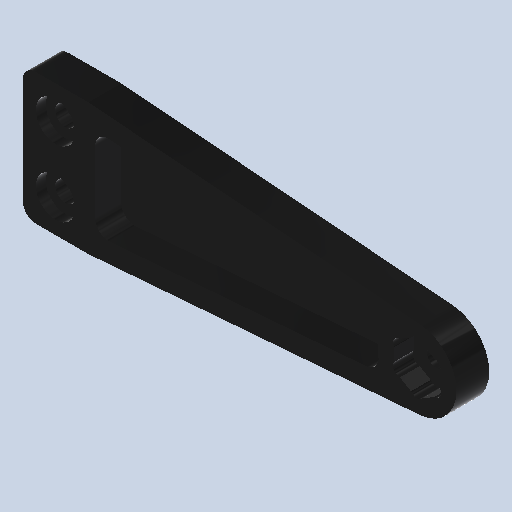
# Autodesk Inventor part: Trunk_handle_frame
Saved by Autodesk Inventor 2022.4 (Build 264492000, 492)
## iProperties
Created: 2016-05-25
Part Number: Trunk_handle_frame
Material: アセタール樹脂、黒
Document SubType Name: Modeling
Designer: hiroaki
Density: 1.425 g/cm^3
Appearance: 滑らか - 黒
Mass: 4.5833 g
Surface Area: 34.8824 cm^2
Volume: 3.21635 cm^3
Description: POM T5
Author: hiroaki
Autodesk Inventor part; units mm, degrees
ref_plane "YZ Plane" through (0, 0, 0) normal (1, 0, 0) x (0, 1, 0)
ref_plane "XZ Plane" through (0, 0, 0) normal (0, 1, 0) x (-1, 0, 0)
ref_plane "XY Plane" through (0, 0, 0) normal (0, 0, 1) x (1, 0, 0)
sketch "スケッチ1" plane through (0, 0, 0) normal (0, 0, 1) x (1, 0, 0)
  circle A0 centre (5, 5) radius 1.55
  circle A1 centre (5, -5) radius 1.55
  line L0 (0, 0) -> (60, 0) construction
  circle A2 centre (60, 0) radius 1.55
  line L1 (0, 10) -> (0, -10)
  line L2 (0, -10) -> (10, -10)
  line L3 (10, -10) -> (60.4762, -5.9811)
  line L4 (10, 10) -> (60.4762, 5.9811)
  arc A3 (60.4762, -5.9811) -> (60.4762, 5.9811) centre (60, 0) ccw
  line L5 (55.0583, -3.4029) -> (11, -6.9109)
  line L6 (55.0583, 3.4029) -> (11, 6.9109)
  arc A4 (55.0583, 3.4029) -> (55.0583, -3.4029) centre (60, 0) ccw
  line L7 (11, -6.9109) -> (11, 6.9109)
  line L8 (5, -5) -> (5, 5) construction
  line L9 (0, 10) -> (10, 10)
  line L10 (8.01, 6.7378) -> (8.01, 3.2622) construction
  line L11 (8.01, 3.2622) -> (5, 1.5244) construction
  line L12 (5, 1.5244) -> (1.99, 3.2622) construction
  line L13 (1.99, 3.2622) -> (1.99, 6.7378) construction
  line L14 (1.99, 6.7378) -> (5, 8.4756) construction
  line L15 (5, 8.4756) -> (8.01, 6.7378) construction
  arc A5 (4.0907, 2.0494) -> (5.9093, 2.0494) centre (5, 2.5744) ccw construction
  arc A6 (7.1007, 2.7372) -> (8.01, 4.3122) centre (7.1007, 3.7872) ccw construction
  arc A7 (8.01, 5.6878) -> (7.1007, 7.2628) centre (7.1007, 6.2128) ccw construction
  arc A8 (5.9093, 7.9506) -> (4.0907, 7.9506) centre (5, 7.4256) ccw construction
  arc A9 (2.8993, 7.2628) -> (1.99, 5.6878) centre (2.8993, 6.2128) ccw construction
  arc A10 (1.99, 4.3122) -> (2.8993, 2.7372) centre (2.8993, 3.7872) ccw construction
  line L16 (8.01, -6.7378) -> (8.01, -3.2622) construction
  line L17 (8.01, -3.2622) -> (5, -1.5244) construction
  line L18 (5, -1.5244) -> (1.99, -3.2622) construction
  line L19 (1.99, -3.2622) -> (1.99, -6.7378) construction
  line L20 (1.99, -6.7378) -> (5, -8.4756) construction
  line L21 (5, -8.4756) -> (8.01, -6.7378) construction
  arc A11 (5.9093, -2.0494) -> (4.0907, -2.0494) centre (5, -2.5744) ccw construction
  arc A12 (8.01, -4.3122) -> (7.1007, -2.7372) centre (7.1007, -3.7872) ccw construction
  arc A13 (7.1007, -7.2628) -> (8.01, -5.6878) centre (7.1007, -6.2128) ccw construction
  arc A14 (4.0907, -7.9506) -> (5.9093, -7.9506) centre (5, -7.4256) ccw construction
  arc A15 (1.99, -5.6878) -> (2.8993, -7.2628) centre (2.8993, -6.2128) ccw construction
  arc A16 (2.8993, -2.7372) -> (1.99, -4.3122) centre (2.8993, -3.7872) ccw construction
  circle A17 centre (60, 0) radius 1.55
  line L22 (63.51, 2.0265) -> (63.51, -2.0265)
  line L23 (63.51, -2.0265) -> (60, -4.053)
  line L24 (60, -4.053) -> (56.49, -2.0265)
  line L25 (56.49, -2.0265) -> (56.49, 2.0265)
  line L26 (56.49, 2.0265) -> (60, 4.053)
  line L27 (60, 4.053) -> (63.51, 2.0265)
  arc A18 (59.0907, -3.528) -> (60.9093, -3.528) centre (60, -3.003) ccw
  arc A19 (62.6007, -2.5515) -> (63.51, -0.9765) centre (62.6007, -1.5015) ccw
  arc A20 (63.51, 0.9765) -> (62.6007, 2.5515) centre (62.6007, 1.5015) ccw
  arc A21 (60.9093, 3.528) -> (59.0907, 3.528) centre (60, 3.003) ccw
  arc A22 (57.3993, 2.5515) -> (56.49, 0.9765) centre (57.3993, 1.5015) ccw
  arc A23 (56.49, -0.9765) -> (57.3993, -2.5515) centre (57.3993, -1.5015) ccw
  line L28 (60, 4.053) -> (60, -4.053) construction
  circle A24 centre (5, 5) radius 3.005
  circle A25 centre (5, -5) radius 3.005
  point P0 (5, 0)
  point P1 (8.01, 3.2622)
  point P2 (8.01, 6.7378)
  point P3 (5, 8.4756)
  point P4 (1.99, 6.7378)
  point P5 (2.8993, 2.7372)
  point P6 (1.99, 4.3122)
  point P7 (1.99, 5.6878)
  point P8 (2.8993, 7.2628)
  point P9 (4.0907, 7.9506)
  point P10 (5.9093, 7.9506)
  point P11 (7.1007, 7.2628)
  point P12 (8.01, 5.6878)
  point P13 (8.01, 4.3122)
  point P14 (7.1007, 2.7372)
  point P15 (7.1007, -2.7372)
  point P16 (8.01, -4.3122)
  point P17 (8.01, -5.6878)
  point P18 (7.1007, -7.2628)
  point P19 (5.9093, -7.9506)
  point P20 (4.0907, -7.9506)
  point P21 (2.8993, -7.2628)
  point P22 (1.99, -5.6878)
  point P23 (1.99, -4.3122)
  point P24 (2.8993, -2.7372)
  point P25 (1.99, -6.7378)
  point P26 (5, -8.4756)
  point P27 (56.49, 2.0265)
  point P28 (56.49, -2.0265)
  point P29 (62.6007, -2.5515)
  point P30 (57.3993, -2.5515)
  point P31 (56.49, -0.9765)
  point P32 (56.49, 0.9765)
  point P33 (57.3993, 2.5515)
  point P34 (59.0907, 3.528)
  point P35 (60.9093, 3.528)
  point P36 (62.6007, 2.5515)
  point P37 (63.51, 0.9765)
  point P38 (63.51, -0.9765)
  dimension "d0" = 10
  dimension "d1" = 3.1
  dimension "d2" = 3.1
  dimension "d3" = 60
  dimension "d4" = 6
  dimension "d33" = 3
  dimension "d34" = 6
  dimension "d35" = 6
  dimension "d40" = 20
  dimension "d41" = 5
  dimension "d42" = 10
  dimension "d43" = 6.02
  dimension "d44" = 2.1
  dimension "d47" = 360
  dimension "d57" = 3.1
  dimension "d58" = 7.02
  dimension "d59" = 2.1
  dimension "d60" = 360
  dimension "d62" = 6.01
  constraints: 58 end point, 53 point on circle, 28 symmetric about line, 26 centre point, 9 point on line, 5 coincident, 3 midpoint, 3 vertical, 2 parallel, 2 perpendicular, 2 tangent, 1 concentric, 1 equal radius, 1 horizontal, 95 other
  measures "d0" distance of L8.end L8.start
  measures "d1" diameter of A0
  measures "d2" diameter of A2
  measures "d3" distance of L0.end L0.start
  measures "d4" radius of A3
  measures "d33" distance between parallel lines of L3 L5
  measures "d34" radius of A4
  measures "d35" distance from line of L7 L8.end
  measures "d40" distance of L1.start L1.end
  measures "d41" distance from line of L1 L8.start
  measures "d42" distance of L1.end L2.end
  measures "d43" distance between parallel lines of L13 L10
  measures "d44" diameter of A5
  measures "d57" diameter of A17
  measures "d58" distance between parallel lines of L25 L22
  measures "d59" diameter of A18
  measures "d62" diameter of A24
extrude "押し出し1" add sketch "スケッチ1" along normal blind 5 contours L9 L4 A3 L3 L2 L1
extrude "押し出し5" add sketch "スケッチ1" along normal blind 3.5 contours A24 | A25
extrude "押し出し6" add sketch "スケッチ1" along normal blind 2 contours A20 L22 | L22 L23 L24 L25 L26 L27 | L27 A20 | A19 L22 | L27 A21 | A19 L23 | L26 A21 | A18 L23 | L26 A22 | A18 L24 | L25 A22 | A23 L24 | L25 A23
extrude "押し出し7" add sketch "スケッチ1" along normal blind 1 contours L5 L7 L6 A4
fillet "フィレット2" radius 2 6 edges at (11, 6.9109, 3) (11, -6.9109, 3) (55.0583, 3.4029, 3) (55.0583, -3.4029, 3) (0, -10, 2.5) (0, 10, 2.5)
